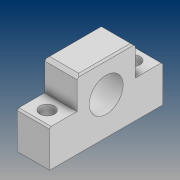
# Autodesk Inventor part: Goi_do_A
Saved by Autodesk Inventor 2021 (Build 250183000, 183)
## iProperties
Created: 2024-04-08
Part Number: Goi_do_A
Material: Generic
Document SubType Name: Modeling
Designer: Admin
Density: 1 g/cm^3
Appearance: Default
Author: Admin
Autodesk Inventor part; units mm, degrees
ref_plane "YZ Plane" through (0, 0, 0) normal (1, 0, 0) x (0, 1, 0)
ref_plane "XZ Plane" through (0, 0, 0) normal (0, 1, 0) x (-1, 0, 0)
ref_plane "XY Plane" through (0, 0, 0) normal (0, 0, 1) x (1, 0, 0)
sketch "Sketch1" plane through (0, 0, 0) normal (1, 0, 0) x (0, 1, 0)
  line L0 (-24, 35) -> (24, 35)
  line L1 (24, 35) -> (24, -35)
  line L2 (24, -35) -> (-24, -35)
  line L3 (-24, -35) -> (-24, 35)
  line L4 (-24, 35) -> (24, -35) construction
  line L5 (24, 35) -> (-24, -35) construction
  line L6 (-43, 18) -> (43, 18)
  line L7 (43, 18) -> (43, -18)
  line L8 (43, -18) -> (-43, -18)
  line L9 (-43, -18) -> (-43, 18)
  line L10 (-43, 18) -> (43, -18) construction
  line L11 (43, 18) -> (-43, -18) construction
  circle A0 centre (24, 0) radius 10.5
  line L12 (0, 35) -> (0, -35)
  point P0 (0, 0)
  point P1 (24, -18)
  point P2 (24, 18)
  dimension "d0" = 36
  dimension "d1" = 70
  dimension "d2" = 19
  dimension "d3" = 24
  dimension "d4" = 21
  constraints: 26 end point, 7 midpoint, 4 parallel, 2 horizontal, 2 perpendicular, 1 centre point
  measures "d0" distance between parallel lines of L6 L8
  measures "d1" distance between parallel lines of L0 L2
  measures "d2" distance between parallel lines of L7 L1
  measures "d3" distance from line of point (0, 0) L1
  measures "d4" diameter of A0
extrude "Extrusion1" add sketch "Sketch1" along normal mid plane 20 contours L0 L1 L6 L12 | L6 L1 A0 L8 L12 | L6 L7 L8 L1 A0 | L8 L1 L2 L12
sketch "Sketch2" plane through (-10, 24, -18) normal (0, 1, 0) x (1, 0, 0)
  line L0 (0, 0) -> (20, 0) projected
  line L1 (20, 17) -> (20, 0) projected
  line L2 (0, 17) -> (20, 17) projected
  line L3 (0, 0) -> (0, 17) projected
  line L4 (0, -53) -> (20, -53) projected
  line L5 (20, -36) -> (20, -53) projected
  line L6 (0, -36) -> (20, -36) projected
  line L7 (0, -53) -> (0, -36) projected
  line L8 (0, -53) -> (20, -36)
  line L9 (20, 17) -> (20, 0) projected
  line L10 (20, 0) -> (0, 17)
  point P0 (10, -18)
  point P1 (10, -44.5)
  point P2 (10, 8.5)
  constraints: 4 end point, 2 midpoint
hole "Hole1" at (0, 24, 26.5) at (0, 24, -26.5) direction (0, -1, 0) diameter 9 end through all
chamfer "Chamfer1" distance 1 angle 45 2 edges at (-10, 43, 0) (10, 43, 0)
chamfer "Chamfer2" distance 1 angle 45 6 edges at (0, 24, 35) (0, 24, -35) (-10, 0, 0) (0, 0, -35) (10, 0, 0) (0, 0, 35)
chamfer "Chamfer3" distance 2 angle 45 2 edges at (0, 43, -18) (0, 43, 18)
body "Solid1"
